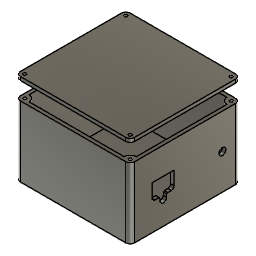
CheeseMaker-ElectricsCase v5 (Autodesk Fusion 360 design; units mm, degrees)
Autodesk Fusion 360 part; units mm, degrees
sketch "Sketch1" plane through (0, 0, 0) normal (0, 0, 1) x (1, 0, 0)
  line L0 (0, 0) -> (-130, 0)
  line L1 (-130, 0) -> (-130, 125)
  line L2 (-130, 125) -> (0, 125)
  line L3 (0, 125) -> (0, 0)
  line L4 (-4, 4) -> (-126, 4)
  line L5 (-126, 4) -> (-126, 121)
  line L6 (-126, 121) -> (-4, 121)
  line L7 (-4, 121) -> (-4, 4)
  line L8 (-126, 4) -> (-55, 4)
  line L9 (-55, 4) -> (-55, 56)
  line L10 (-55, 56) -> (-126, 56)
  line L11 (-126, 56) -> (-126, 4)
  line L12 (-126, 56) -> (-55, 56)
  line L13 (-55, 56) -> (-55, 25)
  line L14 (-55, 25) -> (-126, 25)
  line L15 (-126, 25) -> (-126, 56)
  line L16 (-126, 25) -> (-114.5, 25)
  circle A0 centre (-114.5, 25) radius 2.4
  line L17 (-114.5, 25) -> (-67, 25)
  circle A1 centre (-67, 25) radius 2.4
  line L18 (-126, 56) -> (-126, 61)
  line L19 (-126, 61) -> (-24, 61)
  line L20 (-24, 61) -> (-24, 114.5)
  line L21 (-24, 114.5) -> (-126, 114.5)
  line L22 (-126, 114.5) -> (-126, 61)
  line L23 (-126, 114.5) -> (-126, 111.8)
  line L24 (-126, 111.8) -> (-122, 111.8)
  circle A2 centre (-122, 111.8) radius 1.55
  line L25 (-122, 111.8) -> (-39.5, 111.8)
  circle A3 centre (-39.5, 111.8) radius 1.55
  line L26 (-122, 111.8) -> (-122, 78.8)
  line L27 (-122, 78.8) -> (-91, 78.8)
  circle A4 centre (-91, 78.8) radius 1.55
  dimension "d1" = 130
  dimension "d2" = 125
  dimension "d3" = 4
  dimension "d25" = 71
  dimension "d26" = 52
  dimension "d43" = 11.5
  dimension "d44" = 4.8
  dimension "d45" = 47.5
  dimension "d46" = 4.8
  dimension "d49" = 5
  dimension "d50" = 102
  dimension "d51" = 53.5
  dimension "d52" = 2.7
  dimension "d53" = 4
  dimension "d54" = 3.1
  dimension "d55" = 82.5
  dimension "d56" = 3.1
  dimension "d57" = 33
  dimension "d58" = 90
  dimension "d59" = 31
  dimension "d60" = 3.1
  constraint horizontal L0
  constraint vertical L1
  constraint horizontal L2
  constraint vertical L3
  constraint coincident L0.start L3.end
  constraint horizontal L8
  constraint vertical L9
  constraint horizontal L10
  constraint vertical L11
  constraint horizontal L12
  constraint vertical L13
  constraint horizontal L14
  constraint vertical L15
  constraint coincident L9 L13.end
  constraint horizontal L16
  constraint coincident L16.end A0.centre
  constraint horizontal L17
  constraint coincident L17.end A1.centre
  constraint vertical L18
  constraint horizontal L19
  constraint vertical L20
  constraint horizontal L21
  constraint vertical L22
  constraint vertical L23
  constraint horizontal L24
  constraint coincident L24.end A2.centre
  constraint horizontal L25
  constraint coincident L25.end A3.centre
  constraint perpendicular L25 L26
  constraint coincident L27.end A4.centre
  measures "d1" distance of L0.start L0.end
  measures "d2" distance of L0.start L2.end
  measures "d25" distance of L4.end L8.end
  measures "d26" distance of L4.end L10.end
  measures "d43" distance of L14.end L16.end
  measures "d44" diameter of A0
  measures "d45" distance of L16.end L17.end
  measures "d46" diameter of A1
  measures "d49" distance of L10.end L18.end
  measures "d50" distance of L18.end L19.end
  measures "d51" distance of L18.end L21.end
  measures "d52" distance of L21.end L23.end
  measures "d53" distance of L23.end L24.end
  measures "d54" diameter of A2
  measures "d55" distance of L24.end L25.end
  measures "d56" diameter of A3
  measures "d57" distance of L24.end L26.end
  measures "d58" angle of L26 L27
  measures "d59" distance of L26.end L27.end
  measures "d60" diameter of A4
extrude "Extrude1" add sketch "Sketch1" along normal blind 80 contours L0 L1 L2 L3 makes body 1
extrude "Extrude2" add sketch "Sketch1" along normal blind 4 contours L4 L5 L6 L7 L9 L10 L12 L13 L18 L19 L20 L21 | L4 L5 L8 L9 L11 L14 L16 A0 L17 A1 | L5 L9 L10 L11 L12 L13 L14 L15 L16 A0 L17 A1 | L14 L17 A1 | L14 L17 A1 | L5 L19 L20 L21 L22 L23 | L14 L16 A0 L17 | L14 L16 A0 L17 | L24 A2 L25 | L24 A2 L26 | A2 L25 L26 | A3 | A4 bodies 1
sketch "Sketch2" plane through (0, 0, 80) normal (0, 0, 1) x (-1, 0, 0)
  line L0 (126, -121) -> (4, -121)
  line L1 (4, -121) -> (4, -4)
  line L2 (4, -4) -> (126, -4)
  line L3 (126, -4) -> (126, -121)
  line L4 (0, -125) -> (130, -125)
  line L5 (130, -125) -> (130, 0)
  line L6 (130, 0) -> (0, 0)
  line L7 (0, 0) -> (0, -125)
  circle A0 centre (126, -121) radius 7
  circle A1 centre (4, -121) radius 7
  circle A2 centre (4, -4) radius 7
  circle A3 centre (126, -4) radius 7
  circle A4 centre (126, -4) radius 1.8
  circle A5 centre (4, -4) radius 1.8
  circle A6 centre (4, -121) radius 1.8
  circle A7 centre (126, -121) radius 1.8
  dimension "d9" = 14
  dimension "d10" = 14
  dimension "d11" = 14
  dimension "d12" = 14
  dimension "d65" = 3.6
  dimension "d66" = 3.6
  dimension "d67" = 3.6
  dimension "d68" = 3.6
  constraint coincident L0.start L3.end
  constraint coincident L0.end L1.start
  constraint coincident L1.end L2.start
  constraint coincident L2.end L3.start
  constraint concentric A0 A7
  measures "d9" diameter of A0
  measures "d10" diameter of A1
  measures "d11" diameter of A2
  measures "d12" diameter of A3
  measures "d65" diameter of A4
  measures "d66" diameter of A5
  measures "d67" diameter of A6
  measures "d68" diameter of A7
extrude "Extrude3" add sketch "Sketch2" against normal blind 10 contours L0 L1 A1 A6 | L0 L1 A6 | L0 L3 A0 A7 | L0 L3 A7 | L1 L2 A2 A5 | L2 L3 A3 A4 | L1 L2 A5 | L2 L3 A4 picked at (4.9582, -120.2827) picked at (125.1536, -120.1536) picked at (5.1215, -4.4183) picked at (125.7456, -5.1696) bodies 1
sketch "Sketch3" plane through (0, 0, 80) normal (0, 0, 1) x (-1, 0, 0)
  line L0 (119, -121) -> (11, -121)
  arc A0 (11, -121) -> (4, -114) centre (4, -121) ccw
  line L1 (4, -114) -> (4, -11)
  arc A1 (4, -11) -> (11, -4) centre (4, -4) ccw
  line L2 (11, -4) -> (119, -4)
  arc A2 (119, -4) -> (126, -11) centre (126, -4) ccw
  line L3 (126, -11) -> (126, -114)
  arc A3 (126, -114) -> (119, -121) centre (126, -121) ccw
  line L4 (0, -125) -> (130, -125)
  line L5 (130, -125) -> (130, 0)
  line L6 (130, 0) -> (0, 0)
  line L7 (0, 0) -> (0, -125)
extrude "Extrude4" add sketch "Sketch3" along normal blind 4 separate body makes body 2
extrude "Extrude5" add sketch "Sketch3" along normal blind 4 separate body contours L0 A0 L1 A1 L2 A2 L3 A3 makes body 3
extrude "Extrude6" add sketch "Sketch3" against normal blind 4 contours L0 A0 L1 A1 L2 A2 L3 A3 bodies 3 2
sketch "Sketch4" plane through (0, 0, 0) normal (1, 0, 0) x (0, 1, 0)
  line L0 (0, 0) -> (125, 0)
  line L1 (125, 0) -> (125, 80)
  line L2 (125, 80) -> (0, 80)
  line L3 (0, 80) -> (0, 0)
  line L4 (0, 40) -> (125, 40)
  circle A0 centre (105, 40) radius 3.95
  line L5 (25, 40) -> (50, 40)
  line L6 (50, 40) -> (50, 49.3)
  line L7 (50, 49.3) -> (25, 49.3)
  line L8 (25, 49.3) -> (25, 40)
  line L9 (25, 40) -> (50, 40)
  line L10 (50, 40) -> (50, 30.7)
  line L11 (50, 30.7) -> (25, 30.7)
  line L12 (25, 30.7) -> (25, 40)
  circle A1 centre (37.7408, 26.85) radius 3.85
  line L13 (41.5908, 26.844) -> (41.5968, 30.7)
  line L14 (33.8908, 26.844) -> (33.8848, 30.7)
  dimension "d21" = 7.9
  dimension "d22" = 20
  dimension "d27" = 9.3
  dimension "d28" = 25
  dimension "d29" = 9.3
  dimension "d30" = 7.7
  constraint midpoint L3 L4.start
  constraint midpoint L1 L4.end
  constraint coincident L4 A0.centre
  constraint horizontal L5
  constraint vertical L6
  constraint horizontal L7
  constraint vertical L8
  constraint coincident L4 L5.start
  constraint horizontal L9
  constraint vertical L10
  constraint horizontal L11
  constraint vertical L12
  constraint tangent L11 A1
  constraint coincident A1 L13.start
  constraint coincident L11 L13.end
  constraint tangent A1 L13
  constraint coincident A1 L14.start
  constraint coincident L11 L14.end
  constraint tangent A1 L14
  measures "d21" diameter of A0
  measures "d22" distance of L4.end A0.centre
  measures "d27" distance of L5.start L7.end
  measures "d28" distance of L5.start L5.end
  measures "d29" distance of L5.start L11.end
  measures "d30" diameter of A1
extrude "Extrude7" cut sketch "Sketch4" against normal up to surface (4 mm away) contours L4 L5 L6 L7 L8 L9 | L4 L5 L9 L10 L11 L12 | L4 A0 | L4 A0 | L11 A1 L14 | L11 A1 L13 | A1 L13 bodies 1
sketch "Sketch5" plane through (-130, 0, 0) normal (-1, 0, 0) x (0, -1, 0)
  line L0 (-125, 0) -> (0, 0)
  line L1 (0, 0) -> (0, 80)
  line L2 (0, 80) -> (-125, 80)
  line L3 (-125, 80) -> (-125, 0)
  line L4 (-125, 80) -> (0, 80)
  line L5 (0, 80) -> (0, 40)
  line L6 (0, 40) -> (-125, 40)
  line L7 (-125, 40) -> (-125, 80)
  circle A0 centre (-95, 40) radius 4
  circle A1 centre (-81, 40) radius 4
  circle A2 centre (-67, 40) radius 4
  line L8 (-32.7193, 40) -> (-18.7193, 40)
  line L9 (-18.7193, 40) -> (-18.7193, 42.7)
  line L10 (-18.7193, 42.7) -> (-32.7193, 42.7)
  line L11 (-32.7193, 42.7) -> (-32.7193, 40)
  line L12 (-32.7193, 40) -> (-18.7193, 40)
  line L13 (-18.7193, 40) -> (-18.7193, 37.3)
  line L14 (-18.7193, 37.3) -> (-32.7193, 37.3)
  line L15 (-32.7193, 37.3) -> (-32.7193, 40)
  dimension "d31" = 8
  dimension "d32" = 8
  dimension "d33" = 8
  dimension "d34" = 14
  dimension "d35" = 2.7
  dimension "d36" = 14
  dimension "d37" = 2.7
  dimension "d38" = 30
  dimension "d39" = 14
  dimension "d40" = 14
  constraint horizontal L4
  constraint vertical L5
  constraint horizontal L6
  constraint vertical L7
  constraint midpoint L1 L5.end
  constraint coincident L2.end L3.start
  constraint coincident L6 A0.centre
  constraint coincident L6 A1.centre
  constraint coincident L6 A2.centre
  constraint horizontal L8
  constraint vertical L9
  constraint horizontal L10
  constraint vertical L11
  constraint coincident L6 L8.start
  constraint horizontal L12
  constraint vertical L13
  constraint horizontal L14
  constraint vertical L15
  measures "d31" diameter of A0
  measures "d32" diameter of A1
  measures "d33" diameter of A2
  measures "d34" distance of L8.start L8.end
  measures "d35" distance of L8.start L10.end
  measures "d36" distance of L8.start L8.end
  measures "d37" distance of L8.start L14.end
  measures "d38" distance of L6.end A0.centre
  measures "d39" distance of A0.centre A1.centre
  measures "d40" distance of A1.centre A2.centre
extrude "Extrude8" cut sketch "Sketch5" against normal up to surface (4 mm away) contours L6 A0 | L6 A0 | L6 L8 L12 L13 L14 L15 | L6 L8 L9 L10 L11 L12 | L6 A1 | L6 A1 | L6 A2 | L6 A2 bodies 1
extrude "Extrude9" cut sketch "Sketch1" along normal up to surface (4 mm away) contours L14 L17 A1 | L14 L17 A1 | L14 L16 A0 L17 | L14 L16 A0 L17 | L24 A2 L25 | L24 A2 L26 | A2 L25 L26 | A3 | A4 bodies 1
fillet "Fillet1" radius 1 2 edges at (-2, 33.8848, 30.7) (-2, 41.5968, 30.7) on bodies 1
fillet "Fillet2" radius 3 2 edges at (-2, 25, 30.7) (-2, 50, 30.7) on bodies 1
fillet "Fillet3" radius 5 4 edges at (-130, 125, 40) (0, 125, 40) (0, 0, 40) (-130, 0, 40) on bodies 1
fillet "Fillet4" radius 5 4 edges at (-130, 0, 82) (0, 0, 82) (0, 125, 82) (-130, 125, 82) on bodies 2 3
sketch "Sketch6" plane through (0, 0, 80) normal (0, 0, 1) x (-1, 0, 0)
  arc A0 (130, -5) -> (125, 0) centre (125, -5) ccw
  line L0 (125, 0) -> (5, 0)
  arc A1 (5, 0) -> (0, -5) centre (5, -5) ccw
  line L1 (0, -5) -> (0, -120)
  arc A2 (0, -120) -> (5, -125) centre (5, -120) ccw
  line L2 (5, -125) -> (125, -125)
  arc A3 (125, -125) -> (130, -120) centre (125, -120) ccw
  line L3 (130, -120) -> (130, -5)
  line L4 (119, -121) -> (11, -121)
  arc A4 (11, -121) -> (4, -114) centre (4, -121) ccw
  line L5 (4, -114) -> (4, -11)
  arc A5 (4, -11) -> (11, -4) centre (4, -4) ccw
  line L6 (11, -4) -> (119, -4)
  arc A6 (119, -4) -> (126, -11) centre (126, -4) ccw
  line L7 (126, -11) -> (126, -114)
  arc A7 (126, -114) -> (119, -121) centre (126, -121) ccw
  circle A8 centre (125, -120) radius 1.8
  circle A9 centre (5, -120) radius 1.8
  circle A10 centre (125, -5) radius 1.8
  circle A11 centre (5, -5) radius 1.8
  dimension "d69" = 3.6
  dimension "d72" = 3.6
  dimension "d73" = 3.6
  dimension "d74" = 3.6
  constraint concentric A3 A8
  constraint concentric A2 A9
  constraint concentric A0 A10
  constraint concentric A1 A11
  measures "d69" diameter of A8
  measures "d72" diameter of A9
  measures "d73" diameter of A10
  measures "d74" diameter of A11
extrude "Extrude10" cut sketch "Sketch6" against normal blind 8 contours A8 | A9 | A10 | A11 bodies 1
thread "Thread1" "ISO Metric profile 4.0 M4x0.7 6H" major diameter 4.1095 minor diameter 3.332 pitch 0.7 angle 60 resizes the face on face at (-125.0449, 118.2006, 74.6667) on bodies 1
thread "Thread2" "ISO Metric profile 4.0 M4x0.7 6H" major diameter 4.1095 minor diameter 3.332 pitch 0.7 angle 60 resizes the face on face at (-6.3789, 118.843, 74.6667) on bodies 1
thread "Thread3" "ISO Metric profile 4.0 M4x0.7 6H" major diameter 4.1095 minor diameter 3.332 pitch 0.7 angle 60 resizes the face on face at (-6.7978, 5.0897, 74.6667) on bodies 1
thread "Thread4" "ISO Metric profile 4.0 M4x0.7 6H" major diameter 4.1095 minor diameter 3.332 pitch 0.7 angle 60 resizes the face on face at (-123.7432, 3.7114, 74.6667) on bodies 1
extrude "Extrude11" cut sketch "Sketch6" along normal up to surface (4 mm away) contours A8 | A9 | A10 | A11 bodies 3
move_body "Move1" bodies 3 to x (1, 0, 0) y (0, 1, 0) z (0, 0, 1) at (0, 0, 20)
sketch "Sketch7" plane through (0, 0, 96) normal (0, 0, -1) x (1, 0, 0)
  line L0 (-126, -11) -> (-126, -114)
  arc A0 (-119, -121) -> (-126, -114) centre (-126, -121) ccw
  line L1 (-119, -121) -> (-11, -121)
  arc A1 (-4, -114) -> (-11, -121) centre (-4, -121) ccw
  line L2 (-4, -114) -> (-4, -11)
  arc A2 (-11, -4) -> (-4, -11) centre (-4, -4) ccw
  line L3 (-11, -4) -> (-119, -4)
  arc A3 (-126, -11) -> (-119, -4) centre (-126, -4) ccw
  arc A4 (-118.5167, -120.5) -> (-125.5, -113.5167) centre (-126, -121) ccw
  line L4 (-125.5, -11.4833) -> (-125.5, -113.5167)
  arc A5 (-125.5, -11.4833) -> (-118.5167, -4.5) centre (-126, -4) ccw
  line L5 (-11.4833, -4.5) -> (-118.5167, -4.5)
  arc A6 (-11.4833, -4.5) -> (-4.5, -11.4833) centre (-4, -4) ccw
  line L6 (-4.5, -113.5167) -> (-4.5, -11.4833)
  arc A7 (-4.5, -113.5167) -> (-11.4833, -120.5) centre (-4, -121) ccw
  line L7 (-118.5167, -120.5) -> (-11.4833, -120.5)
  dimension "d77" = -0.5
extrude "Extrude12" cut sketch "Sketch7" against normal up to surface (4 mm away) bodies 3
equation "d43 = 5 mm + 6.5 mm"
named bodies: "Case", "Lid"
